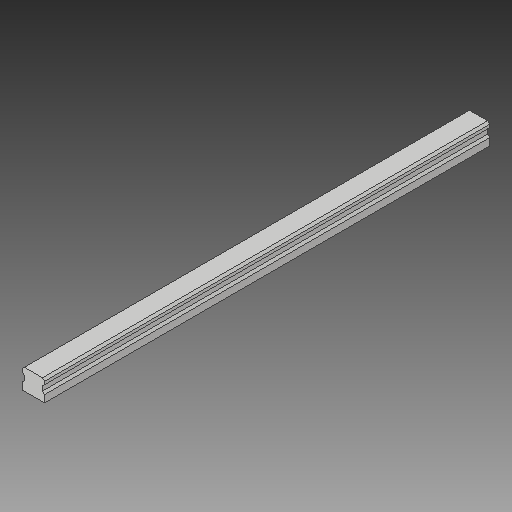
# Autodesk Inventor part: TRILHO LINEAR 15MM DFH-A_AL
Saved by Autodesk Inventor 2018 (Build 220112000, 112)
## iProperties
Created: 2018-09-22
Part Number: TRILHO LINEAR 15MM DFH-A_AL
Material: Genérico
Document SubType Name: Modeling
Designer: Usuario
Density: 1 g/cm^3
Appearance: Padrão
Mass: 58.7913 g
Surface Area: 179.932 cm^2
Volume: 58.7913 cm^3
Author: Usuario
Autodesk Inventor part; units mm, degrees
ref_plane "YZ Plane" through (0, 0, 0) normal (1, 0, 0) x (0, 1, 0)
ref_plane "XZ Plane" through (0, 0, 0) normal (0, 1, 0) x (-1, 0, 0)
ref_plane "XY Plane" through (0, 0, 0) normal (0, 0, 1) x (1, 0, 0)
sketch "Esboço1" plane through (0, 0, 0) normal (0, 0, 1) x (1, 0, 0)
  line L0 (0.6748, 12.626) -> (0.6748, -17.8976) construction
  line L1 (0.6748, 7.7011) -> (-5.4427, 7.7011)
  line L2 (-5.4427, 7.7011) -> (-6.8252, 6.3185)
  line L3 (-6.8252, 6.3185) -> (-6.8252, 4.3185)
  line L4 (-6.8252, 4.3185) -> (-5.4427, 2.936)
  line L5 (-5.4427, 2.936) -> (-5.4427, -0.064)
  line L6 (-5.4427, -0.064) -> (-6.8252, -1.4465)
  line L7 (-6.8252, -1.4465) -> (-6.8252, -6.2989)
  line L8 (-6.8252, -6.2989) -> (0.6748, -6.2989)
  line L9 (0.6748, 7.7011) -> (6.7923, 7.7011)
  line L10 (6.7923, 7.7011) -> (8.1748, 6.3185)
  line L11 (8.1748, 6.3185) -> (8.1748, 4.3185)
  line L12 (8.1748, 4.3185) -> (6.7923, 2.936)
  line L13 (6.7923, 2.936) -> (6.7923, -0.064)
  line L14 (6.7923, -0.064) -> (8.1748, -1.4465)
  line L15 (8.1748, -1.4465) -> (8.1748, -6.2989)
  line L16 (8.1748, -6.2989) -> (0.6748, -6.2989)
  dimension "d11" = 45
  dimension "d12" = 3
  dimension "d13" = 14
  dimension "d14" = 2
  dimension "d15" = 7.5
  constraints: 34 end point, 7 symmetric about line, 6 point on line, 4 perpendicular, 1 horizontal, 1 parallel, 1 vertical
  measures "d11" angle of L2 L1
  measures "d12" distance of L4.end L5.end
  measures "d13" distance between parallel lines of L8 L1
  measures "d14" distance of L2.end L3.end
  measures "d15" distance of L7.end L8.end
extrude "Extrusão1" add sketch "Esboço1" along normal blind 300
